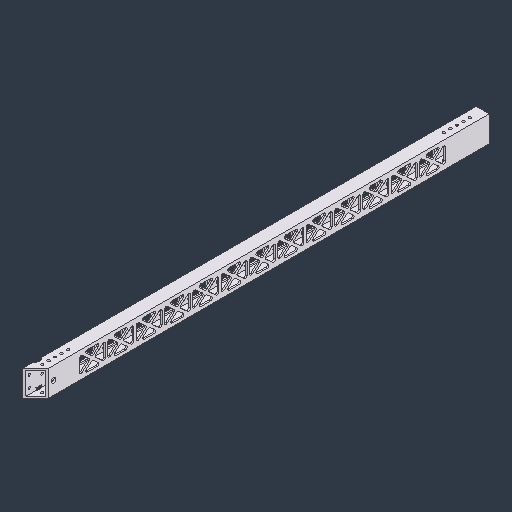
# Autodesk Inventor part: TUBE,ELEVATOR,SIDE,STAGE1
Saved by Autodesk Inventor 2024.3 (Build 283343000, 343)
## iProperties
Created: 2025-01-27
Part Number: TUBE,ELEVATOR,SIDE,STAGE1
Material: Aluminum, 6063-T6
Document SubType Name: Modeling
Designer: Jthib
Density: 2.69879 g/cm^3
Appearance: Metal-AL-6063
Mass: 756.162 g
Surface Area: 2025.44 cm^2
Volume: 280.185 cm^3
Mfg Approved By: John.Thibert
ILogicPurgeVersion: 0.0.0.0
OnSaveVersion: 3.4.3.0
OnSaveAssembly: COREAutomationManager
ModelCat: Uncategorized
MaterialName: Aluminum, 6063-T6
CN_MASS: 1.06
Author: Jthib
Autodesk Inventor part; units mm, degrees
ref_plane "YZ Plane" through (0, 0, 0) normal (1, 0, 0) x (0, 1, 0)
ref_plane "XZ Plane" through (0, 0, 0) normal (0, 1, 0) x (-1, 0, 0)
ref_plane "XY Plane" through (0, 0, 0) normal (0, 0, 1) x (1, 0, 0)
sketch "Sketch1" plane through (0, 0, 0) normal (0, 0, 1) x (1, 0, 0)
  line L0 (-12.7, -25.4) -> (12.7, -25.4)
  line L1 (12.7, -25.4) -> (12.7, 25.4)
  line L2 (12.7, 25.4) -> (-12.7, 25.4)
  line L3 (-12.7, 25.4) -> (-12.7, -25.4)
  line L4 (-12.7, -25.4) -> (12.7, 25.4) construction
  line L5 (12.7, -25.4) -> (-12.7, 25.4) construction
  line L6 (-9.525, 22.225) -> (9.525, 22.225)
  line L7 (9.525, 22.225) -> (9.525, -22.225)
  line L8 (9.525, -22.225) -> (-9.525, -22.225)
  line L9 (-9.525, -22.225) -> (-9.525, 22.225)
  point P0 (0, 0)
  dimension "d0" = 25.4
  dimension "d1" = 50.8
  dimension "d2" = 3.175
  constraints: 20 end point, 4 parallel, 2 midpoint, 2 perpendicular, 1 horizontal, 3 other
  measures "d0" distance of L2.end L1.end
  measures "d1" distance of L1.end L0.end
  measures "d2" distance between parallel lines of L2 L6
extrude "Extrusion1" add sketch "Sketch1" along normal mid plane 889
sketch "Sketch2" plane through (-12.7, -25.4, 444.5) normal (0, -1, 0) x (1, 0, 0)
  line L0 (25.4, 0) -> (25.4, -889) projected
  line L1 (0, 0) -> (25.4, 0) projected
  line L2 (0, -889) -> (0, 0) construction
  line L3 (25.4, -889) -> (0, -889) projected
  line L4 (0, 0) -> (25.4, -25.4)
  line L5 (22.225, 0) -> (3.175, 0) construction
  point P0 (12.7, -444.5)
  dimension "d47" = 45
  constraints: 2 end point, 1 point on line
  measures "d47" angle of L4 L5
extrude "Extrusion2" cut sketch "Sketch2" against normal through all
sketch "Sketch4" plane through (-12.7, -25.4, 444.5) normal (0, -1, 0) x (1, 0, 0)
  line L0 (0, -889) -> (0, 0) construction
  point P0 (12.7, -444.5)
  point P1 (12.7, -76.2)
  point P2 (12.7, -63.5)
  point P3 (12.7, -50.8)
  point P4 (12.7, -38.1)
  point P5 (12.7, -25.4)
  dimension "d9" = 12.7
  dimension "d13" = 12.7
  dimension "d49" = 368.3
  constraints: 1 vertical, 4 other
  measures "d9" distance from line of L0 point (12.7, -76.2)
  measures "d13" distance of point (12.7, -76.2) point (12.7, -63.5)
  measures "d49" distance of point (12.7, -444.5) point (12.7, -76.2)
hole "Hole1" at (0, -25.4, 368.3) at (0, -25.4, 381) at (0, -25.4, 393.7) at (0, -25.4, 406.4) at (0, -25.4, 419.1) direction (0, 1, 0) diameter 5.1054 end through all start extended yes clearance for "Flat Head Machine Screw (82)" size "#10" standard "Ansi Unified Screw Threads"
sketch "Sketch5" plane through (12.7, -25.4, -419.1) normal (1, 0, 0) x (0, 0, -1)
  line L0 (-419.1, 25.4) -> (-828.675, 25.4) construction
  dimension "d25" = 409.575
  constraints: 2 end point, 1 coincident, 1 horizontal
  measures "d25" distance of L0.start L0.end
hole "Hole2" at (12.7, 0, 409.575) direction (-1, 0, 0) diameter 4.9784 end through all counterbore diameter 9.525 counterbore depth 12.7 clearance for "Socket Head Cap Screw" size "#10" standard "Ansi Unified Screw Threads"
sketch "Sketch6" plane through (-9.525, -22.225, -441.325) normal (1, 0, 0) x (0, 0, -1)
  circle A0 centre (-850.9, 22.225) radius 2.4892 construction
  line L0 (-850.9, 22.225) -> (-876.3, 22.225) construction
  line L1 (-876.3, 33.3375) -> (-876.3, 11.1125) construction
  point P0 (-441.325, 22.225)
  dimension "d33" = 25.4
  dimension "d34" = 22.225
  constraints: 4 end point, 1 horizontal, 1 midpoint, 1 vertical
  measures "d33" distance of L0.start L0.end
  measures "d34" distance of L1.start L1.end
hole "Hole3" at (-9.525, -11.1125, 434.975) at (-9.525, 11.1125, 434.975) direction (-1, 0, 0) diameter 4.9784 end through all clearance for "Socket Head Cap Screw" size "#10" standard "Ansi Unified Screw Threads"
sketch "Sketch7" plane through (-12.7, -25.4, -444.5) normal (0, -1, 0) x (1, 0, 0)
  circle A0 centre (-4.7625, 860.425) radius 9.525
  line L0 (0, 0) -> (0, 889) construction
  point P0 (12.7, 444.5)
  dimension "d42" = 4.7625
  dimension "d43" = 28.575
  dimension "d44" = 19.05
  constraints: 1 centre point
  measures "d42" distance from line of L0 A0.centre
  measures "d43" vertical distance of L0.end A0.centre
  measures "d44" diameter of A0
extrude "Extrusion3" cut sketch "Sketch7" against normal blind 7.62
sketch "Sketch8" plane through (12.7, -25.4, -444.5) normal (1, 0, 0) x (0, 0, -1)
  line L0 (-1066.8, 25.4) -> (177.8, 25.4) construction
  line L1 (-444.5, -10.16) -> (-444.5, 60.96) construction
  line L2 (-440.8828, 25.4) -> (-419.1, 44.45)
  line L3 (-419.1, 44.45) -> (-419.1, 6.35)
  line L4 (-419.1, 6.35) -> (-440.8828, 25.4)
  line L5 (-444.5, 28.5634) -> (-426.3344, 44.45)
  line L6 (-426.3344, 44.45) -> (-462.6656, 44.45)
  line L7 (-462.6656, 44.45) -> (-444.5, 28.5634)
  line L8 (-448.1172, 25.4) -> (-469.9, 44.45)
  line L9 (-469.9, 44.45) -> (-469.9, 6.35)
  line L10 (-469.9, 6.35) -> (-448.1172, 25.4)
  line L11 (-444.5, 22.2366) -> (-426.3344, 6.35)
  line L12 (-426.3344, 6.35) -> (-462.6656, 6.35)
  line L13 (-462.6656, 6.35) -> (-444.5, 22.2366)
  point P0 (-444.5, 25.4)
  dimension "d50" = 38.1
  dimension "d51" = 4.7625
  dimension "d52" = 50.8
  constraints: 24 end point, 10 point on line, 2 equal length, 2 parallel, 2 vertical, 1 horizontal, 1 perpendicular, 5 other
  measures "d50" distance between parallel lines of L12 L6
  measures "d51" distance between parallel lines of L2 L5
  measures "d52" distance between parallel lines of L9 L3
extrude "Extrusion4" cut sketch "Sketch8" against normal through all
fillet "Fillet1" radius 3.175 24 edges at (11.1125, 19.05, -25.4) (-11.1125, 19.05, -25.4) (11.1125, 19.05, -18.1656) (-11.1125, 19.05, -18.1656) (-11.1125, -19.05, -25.4) (11.1125, -19.05, -25.4) (-11.1125, -19.05, -18.1656) (11.1125, -19.05, -18.1656) (11.1125, -19.05, 18.1656) (-11.1125, -19.05, 18.1656) (-11.1125, -19.05, 25.4) (11.1125, -19.05, 25.4) (-11.1125, 19.05, 18.1656) (11.1125, 19.05, 18.1656) (11.1125, 19.05, 25.4) (-11.1125, 19.05, 25.4) (11.1125, 0, -3.6172) (-11.1125, 0, -3.6172) (11.1125, -3.1634, 0) (-11.1125, -3.1634, 0) (11.1125, 3.1634, 0) (-11.1125, 3.1634, 0) (-11.1125, 0, 3.6172) (11.1125, 0, 3.6172)
pattern_linear "Rectangular Pattern1" count 13 spacing 55.5625 along (0, 0, 1) of "Extrusion4", "Fillet1" first direction both ways yes
mirror "Mirror2" about plane through (0, 0, 0) normal (0, 1, 0) of "Extrusion3"
mirror "Mirror3" about plane through (0, 0, 0) normal (0, 0, 1) of "Hole1"
body "Solid1"
